Autodesk Fusion 360 part; units mm, degrees
note: some values were not read from the file. Chosen so that the rebuilt part matches the saved one: which pieces of a blend or face edit are solid. Set by a fixed rule: which sketch regions a step uses.
(part 3 of 3)
  dimension "d82" = 12
  dimension "d85" = 54
  dimension "d86" = 46.76
  dimension "d87" = 12
  dimension "d88" = 27
  dimension "d89" = 3
  dimension "d90" = -3
  dimension "d104" = 118
  dimension "d105" = 0
  dimension "d108" = 96
  dimension "d109" = 0
  dimension "d110" = 198
  dimension "d111" = 146
  constraint horizontal L0
  constraint vertical L1
  constraint horizontal L2
  constraint vertical L3
  constraint coincident L0.start L3.end
  constraint coincident L2.end L3.start
  constraint coincident L1.end L2.start
  constraint coincident L0.end L1.start
  constraint coincident L0 P0
  constraint midpoint L3 P6
  constraint midpoint L1 L4.end
  constraint coincident A0 L15.start
  constraint coincident A2 L16.end
  constraint parallel L2 L15
  constraint coincident A3 L17.start
  constraint coincident A1 L18.end
  constraint parallel L0 L17
  constraint concentric A4 A5
  constraint tangent A5 L15
  constraint coincident P6 P1
  constraint horizontal L6
  constraint horizontal L8
  constraint coincident L3 P8
  constraint coincident P8 P3
  constraint horizontal L10
  constraint perpendicular L14 L17
  constraint concentric A1 A6
  constraint concentric A0 A7
  constraint concentric A3 A8
  constraint concentric A2 A9
  constraint collinear L15 L16
  constraint collinear L17 L18
  constraint tangent L13 A10
  constraint tangent L20 A10
  constraint tangent L11 A11
  constraint tangent L19 A11
  constraint tangent L19 A12
  constraint tangent L14 A12
  constraint tangent L20 A13
  constraint tangent L12 A13
  constraint vertical L12
  constraint vertical L11
  constraint horizontal L19
  constraint horizontal L20
  constraint vertical L13
  constraint horizontal L33
  constraint horizontal L45
  constraint horizontal L36
  constraint horizontal L51
  constraint coincident L3 P10
  constraint horizontal L57
  constraint coincident A7 L58.start
  constraint coincident L2 L58.start
  constraint coincident A6 L58.end
  constraint coincident L0 L58.end
  constraint coincident A9 L59.start
  constraint coincident L2 L59.start
  constraint coincident A8 L59.end
  constraint coincident L0 L59.end
  constraint coincident L2 A4.centre
  constraint coincident A5 L15.end
  constraint coincident A5 L13.start
  constraint tangent A5 L13
  constraint coincident L12.start A18
  constraint coincident L18.start A18
  constraint tangent L18 A14
  constraint tangent L11 A16
  constraint coincident L11.start A16
  constraint coincident L14.end A27
  constraint tangent L14 A27
  constraint tangent L12 A18
  constraint perpendicular L1252 L1554
  measures "d1" distance of L0.start L0.end
  measures "d10" diameter of A0
  measures "d11" diameter of A1
  measures "d12" diameter of A2
  measures "d13" diameter of A3
  measures "d16" diameter of A4
  measures "d17" distance of L2 L15
  measures "d18" distance of L0 L17
  measures "d26" angle of L5 L6
  measures "d29" angle of L7 L8
  measures "d31" angle of L9 L10
  measures "d34" distance of P6 P8
  measures "d43" diameter of A6
  measures "d44" diameter of A7
  measures "d45" diameter of A8
  measures "d46" diameter of A9
  measures "d48" radius of A10
  measures "d49" radius of A11
  measures "d50" radius of A12
  measures "d51" radius of A13
  measures "d65" distance of L19 L20
  measures "d66" distance of L4 L19
  measures "d78" distance of L5 P8
  measures "d79" distance of P6 L33
  measures "d81" distance of P8 L45
  measures "d87" distance of P10 L57
  measures "d88" distance of P6 P10
  measures "d110" distance of A4.centre A24.centre
  measures "d111" distance of A4.centre L2.end
extrude "Extrude1" add sketch "Sketch1" along normal blind 14 contours A0 A7 L53 L54 L55 L257 L258 | A0 A1 A5 A14 A18 L21 A20 L22 A21 L23 L24 L25 L28 L29 L30 L33 L43 L44 L45 L46 L49 L50 L51 L52 L53 L57 L61 L70 L72 L73 L77 L78 L79 L81 L82 L90 L91 L92 L257 L260 L261 L263 L310 L312 L313 L314 L316 L317 L318 L319 L320 L321 L322 L323 L324 L330 L331 L332 L333 L334 L342 L346 L482 L483 L484 L492 L493 L494 L495 L496 L497 L501 L502 L503 L511 L512 L513 L514 L521 L522 L523 L525 L527 L528 L529 L530 L531 L532 L533 L540 L541 L542 L543 L544 L545 L549 L550 L551 L559 L560 L561 L562 L563 L564 L565 L568 L569 L570 L571 L733 L734 L781 L782 | A0 L257 L258 | A0 L53 L54 L61 | A0 L57 L58 L61 | A0 L54 L58 L61 | A0 L15 L24 L258 | L15 L24 L258 L260 | A0 A7 L54 L55 L58 | L30 L57 L58 L61 | L15 L24 L260 L484 | L30 L33 L58 L61 | L15 L24 L482 L484 | L24 L482 L483 L484 | L33 L45 L58 L61 | L15 L24 L482 L492 | A1 L45 L58 L61 | L15 L24 L492 L496 | A1 L42 L58 L61 | A1 L42 L43 L61 | L15 L24 L496 L497 | A1 A6 L41 L42 L58 | A1 A6 L41 L42 L43 L46 L47 | L15 L24 L497 L501 | L24 L497 L501 L503 | L15 L24 L501 L502 | A1 L18 L25 L47 | A1 L46 L47 | L15 L24 L502 L514 | L18 L25 L47 L49 | L15 L24 L514 L733 | L18 L25 L49 L77 | A5 L15 L24 L733 | A5 L24 L733 L734 | L18 L25 L73 L77 | A5 L734 L735 | L25 L72 L73 L77 | L18 L25 L73 L79 | A4 A5 L523 L524 L734 L735 L748 L749 | L18 L25 L79 L81 | A4 A5 L21 L523 L524 | L18 L25 L81 L90 | A5 L748 L749 | A5 L21 L524 | A5 L13 L21 L524 L525 | L18 L25 L90 L92 | A5 L13 L748 | A5 L13 L524 L748 | L13 A10 L21 A20 L525 L526 L529 L530 L535 L539 L540 | L25 L90 L91 L92 | L18 L25 L92 L316 | L21 A20 L529 L530 | L18 L25 L314 L316 | L13 L526 L535 | L18 L25 L314 L324 | L18 A14 L25 L324 | L20 A10 A20 L22 L539 L540 L544 | A14 L25 L323 L324 | L18 A14 L328 | A14 L25 L328 | A14 L25 L323 L328 | L18 A14 L25 L328 L329 | A14 L25 L328 | L20 L22 L544 L545 | A14 A15 L25 L320 L321 L323 L328 L329 L330 | L18 L25 L329 L333 | L20 L22 L545 L549 | A14 A15 L320 L321 | L18 L25 L333 L334 | A14 L329 L330 | L20 L22 L549 L550 | L18 L25 L334 L346 | L20 L22 L550 L562 | L18 L25 L346 L565 | L25 L334 L342 L346 | L20 L22 A21 L562 L781 | L18 A18 L25 L565 L567 | L18 A18 L567 L581 | L20 A13 A21 L781 L782 | L18 A18 L581 | A18 A19 L567 L568 L569 L575 L576 L581 | A18 L25 L567 | A18 L25 L567 L568 | L12 A13 A21 L23 L571 L782 | A18 L576 L581 | A18 A19 L569 L575 | L12 A18 L23 L571 picked at (-6.11229, 80.063542) picked at (175.409304, 31.163565) picked at (9.778758, 79.397633) picked at (7.933632, 74.992287) picked at (4, 58.820203) picked at (5, 75.333333) picked at (10.599079, 82.625193) picked at (19.628119, 82.333333) picked at (-5.975861, 75.691901) picked at (5, 53) picked at (36.26968, 83.166667) picked at (5, 35) picked at (49.167417, 83.166667) picked at (44.450599, 81.330232) picked at (4, 26) picked at (55.618076, 82.333333) picked at (4, 19.179797) picked at (66.3917, 82.333333) picked at (5, 2.666667) picked at (7.933632, 3.007713) picked at (84.667296, 82.333333) picked at (-5.975861, 2.308099) picked at (-6.11229, -2.063542) picked at (91.117955, 83.166667) picked at (91.215971, 81.330232) picked at (104.019273, 83.166667) picked at (10.599079, -4.625193) picked at (9.779197, -1.402707) picked at (113.157072, 82.333333) picked at (19.629909, -4.333333) picked at (131.429086, 82.333333) picked at (36.276842, -5.166667) picked at (135.442209, 82.541972) picked at (135.774404, 81.215707) picked at (49.170998, -5.166667) picked at (146.135399, 82.977036) picked at (44.455971, -3.333333) picked at (55.618076, -4.333333) picked at (149.896231, 77.792737) picked at (66.395281, -4.333333) picked at (148.132043, 74.135815) picked at (84.678039, -4.333333) picked at (150.909828, 80.139556) picked at (149.702921, 73.587232) picked at (150.333333, 64.44664) picked at (91.125117, -5.166667) picked at (151.864694, 76.222378) picked at (151.66289, 73.358797) picked at (151.166667, 58.828347) picked at (95.840145, -3.333333) picked at (102.381657, -4.333333) picked at (153.210199, 38.425578) picked at (113.157072, -4.333333) picked at (151.272341, 52.490696) picked at (131.443411, -4.333333) picked at (135.452953, -4.541972) picked at (168.596866, 34.833333) picked at (135.784085, -3.225963) picked at (148.44301, -5.712236) picked at (147.961885, -4.878902) picked at (145.285286, -3.334884) picked at (150.408509, -5.531332) picked at (148.457669, -4.647389) picked at (172.809437, 35.666667) picked at (149.900039, 0.194164) picked at (167.429787, -4.333333) picked at (183.397773, 35.666667) picked at (148.759831, 3.822414) picked at (178.208783, -4.333333) picked at (150.910613, -2.147933) picked at (201.302794, 35.666667) picked at (189.463532, -5.166667) picked at (212.938862, 34.833333) picked at (195.907029, -4.333333) picked at (189.368202, -3.334884) picked at (219.573018, 35.666667) picked at (206.011142, -4.333333) picked at (222.378448, -5.338127) picked at (222.749908, 35.617912) picked at (225.276189, -5.974051) picked at (224.39213, -3.81012) picked at (222.490943, -4.235424) picked at (222.706004, -2.592618) picked at (230.333333, 25.663565) picked at (227.183872, -4.892286) picked at (228.47065, 4.015156) picked at (230.333333, 17.618263) makes body 1
extrude "Extrude2" add sketch "Sketch1" along normal blind 14 separate body contours L19 A11 A22 L63 L780 L784 | A11 A22 L770 L780 | L11 A11 L62 A22 L769 L770 | A16 L26 L27 L60 L62 A22 L63 A23 L64 A25 A27 L769 L770 L774 L775 L776 L777 L778 L779 L780 L784 L785 L786 L787 L788 L789 L790 L798 L802 L814 L822 L824 L825 L826 L827 L832 L833 L834 L835 L836 L837 L838 L846 L850 L986 L987 L996 L997 L998 L999 L1000 L1001 L1005 L1006 L1007 L1015 L1016 L1017 L1018 L1019 L1020 L1021 L1023 L1024 L1032 L1033 L1034 L1035 L1036 L1037 L1067 L1068 L1069 L1071 L1072 L1078 L1080 L1081 L1085 L1086 L1087 L1089 L1090 L1098 L1099 L1100 L1237 L1238 L1239 L1249 L1250 L1251 L1252 L1253 L1255 L1256 L1257 L1265 L1266 L1268 L1269 L1271 L1313 L1314 L1324 L1325 L1490 L1491 L1492 L1500 L1501 L1502 L1503 L1504 L1505 L1509 L1510 L1511 L1519 L1524 L1525 | L19 L63 L784 L785 | L11 L62 L769 L775 | L19 L63 L785 L789 | L11 L62 L766 L775 | L19 L63 L789 L790 | L11 A16 L62 L765 L766 | L19 L63 L790 L802 | L11 A16 L765 | A16 L62 L766 | L19 L63 L802 L1021 | A16 L764 L765 | A16 L62 L765 | A16 A17 L62 L764 L765 L766 L774 L987 L988 | A16 A17 L766 L774 | L19 A12 L63 A23 L1021 L1022 L1023 | A16 L27 L988 | L14 A12 A23 L64 L812 L813 L814 L1022 L1023 L1036 L1037 | L16 A16 L27 L986 | A16 L27 L987 L988 | A16 L27 L986 L987 | L16 L27 L986 L996 | L14 L812 L813 | A23 L64 L1036 L1037 | L16 L27 L996 L1000 | L16 L27 L1000 L1001 | L14 L64 A27 L814 L823 | L16 L27 L1001 L1005 | L14 A27 L817 L823 | L16 L27 L1005 L1006 | L27 L1001 L1005 L1007 | L14 A27 L817 | A26 A27 L817 L818 L823 L824 L827 L828 | L64 A27 L823 | L64 A26 A27 L823 L824 | L16 L27 L1006 L1018 | A27 L817 L818 | L16 L27 L1018 L1237 | L16 L27 L1237 L1239 | A27 L827 L828 | L26 A27 L827 L832 | L16 L27 L1239 L1253 | L27 L1237 L1238 L1239 | L17 L26 A27 L832 | L16 L27 A25 L1253 | L17 L26 L832 L833 | L16 L27 A25 L1249 | L27 A25 | L27 A25 L1252 L1253 | L17 L26 L833 L837 | L16 L27 L1249 L1255 | L27 A25 L1252 | L27 A25 L1553 | L17 L26 L837 L838 | L16 L27 L1255 L1257 | A25 L1252 | L17 L26 L838 L850 | L26 L838 L846 L850 | L16 L27 L1257 L1266 | L27 L1255 L1256 L1257 | A25 L1252 L1554 | L17 L26 L850 L1069 | L16 L27 L1266 L1268 | L17 L26 L1069 L1071 | L16 L27 L1268 L1492 | L17 L26 L1071 L1085 | L16 L27 L1490 L1492 | L17 L26 L1081 L1085 | L26 L1080 L1081 L1085 | L16 L27 L1490 L1500 | L27 L1490 L1491 L1492 | L17 L26 L1081 L1087 | L16 L27 L1500 L1504 | L17 L26 L1087 L1089 | L16 L27 L1504 L1505 | L17 L26 L1089 L1098 | L16 L27 L1505 L1509 | L17 L26 L1098 L1100 | L26 L1098 L1099 L1100 | L16 L27 L1509 L1510 | L27 L1505 L1509 L1511 | L17 L26 L1100 L1324 | A2 L16 L27 L1510 | A3 L17 L26 L1324 | A3 L26 L60 L1324 L1325 | A2 | A2 L27 L60 L1510 L1519 | A3 | A3 L59 L60 L1320 L1325 | L59 L60 L1313 L1319 L1320 L1325 | A2 L59 L60 L1519 L1520 | L59 L60 L1519 L1520 L1523 L1524 | L59 L60 L1313 L1314 L1315 L1319 | L59 L60 L1523 L1524 L1525 L1526 | L59 L60 L1314 L1315 L1525 L1526 picked at (240.334724, 42.333333) picked at (223.22752, 45.338574) picked at (220.833333, 55.670564) picked at (223.963533, 57.05587) picked at (248.05205, 42.333333) picked at (221.666667, 59.034158) picked at (254.69695, 43.166667) picked at (221.666667, 66.007755) picked at (267.98675, 43.166667) picked at (220.833333, 69.494553) picked at (276.930307, 42.333333) picked at (220.708473, 73.75994) picked at (223.160749, 71.830131) picked at (293.179806, 43.166667) picked at (222.281583, 78.219094) picked at (221.815094, 74.842155) picked at (223.258231, 75.236965) picked at (225.158818, 73.36066) picked at (299.150792, 43.166667) picked at (227.001287, 83.075443) picked at (316.833333, 19.771431) picked at (238.134749, 82.333333) picked at (228.116601, 81.327131) picked at (237.629901, 81.213143) picked at (244.315389, 83.166667) picked at (316.607755, 25.486044) picked at (314.540637, 39.702424) picked at (253.449606, 82.333333) picked at (270.082214, 83.166667) picked at (317.666667, 13.953212) picked at (282.990695, 83.166667) picked at (316.267565, 4.095355) picked at (291.080761, 83.166667) picked at (282.890888, 81.327131) picked at (316.076333, 1.310426) picked at (317.937429, 0.003905) picked at (318.158468, 4.077407) picked at (319.583407, 3.526062) picked at (300.214978, 82.333333) picked at (316.850928, -1.850259) picked at (316.845795, 83.166667) picked at (329.754276, 83.166667) picked at (319.78146, -4.62039) picked at (331.974842, -3.231092) picked at (336.210307, 82.333333) picked at (329.653574, 81.32558) picked at (332.305449, -4.541972) picked at (339.054767, 82.541972) picked at (336.194191, -4.333333) picked at (358.319413, 82.333333) picked at (345.253104, 81.892093) picked at (337.750223, 80.324153) picked at (354.487693, -4.333333) picked at (363.607586, 83.166667) picked at (340.208322, 75.873434) picked at (349.228141, 81.318612) picked at (363.634445, -5.166667) picked at (376.519648, 83.166667) picked at (339.00265, 75.450039) picked at (376.517857, -5.166667) picked at (371.805516, -3.337985) picked at (382.975679, 82.333333) picked at (376.418946, 81.32558) picked at (341.27419, 72.479258) picked at (382.957773, -4.333333) picked at (393.743931, 82.333333) picked at (401.251275, -4.333333) picked at (410.371167, 83.166667) picked at (410.399816, -5.166667) picked at (423.283229, 83.166667) picked at (423.279648, -5.166667) picked at (423.187004, -3.339536) picked at (429.74105, 82.333333) picked at (423.181632, 81.324029) picked at (429.719563, -4.333333) picked at (440.507512, 82.333333) picked at (440.503931, -4.333333) picked at (457.132957, 83.166667) picked at (457.165188, -5.166667) picked at (470.048601, 83.166667) picked at (470.045019, -5.166667) picked at (469.952376, -3.339536) picked at (476.506422, 82.333333) picked at (469.947004, 81.324029) picked at (476.483144, -4.333333) picked at (479.581758, 82.333333) picked at (479.563852, -4.333333) picked at (478.568078, -2.384954) picked at (484.255191, 83.049067) picked at (478.576136, 80.367896) picked at (484.255191, -5.049067) picked at (485.67961, 10.031337) picked at (486.03159, 11.476739) picked at (485.678714, 67.934547) picked at (486.030695, 65.472087) picked at (486, 21.531456) picked at (486, 48.525253) picked at (485.062286, 39.473638) makes body 2
sketch "Sketch2" plane through (0, -6, 0) normal (0, -1, 0) x (1, 0, 0)
  line L0 (8, 0) -> (226, 0)
  line L1 (226, 0) -> (226, 14)
  line L2 (226, 14) -> (8, 14)
  line L3 (8, 14) -> (8, 0)
  circle A0 centre (328.140012, 4.999995) radius 2.175
  line L4 (324.965012, 4.999995) -> (324.965012, 0)
  circle A1 centre (220.334997, 4.999999) radius 2.175
  line L5 (217.159997, 0) -> (223.509997, 0)
  circle A2 centre (220.334997, 4.999999) radius 1.699995 construction
  line L6 (223.509997, 4.999999) -> (223.509997, 0)
  circle A3 centre (220.334997, 4.999999) radius 3.175
  line L7 (217.159997, 0) -> (217.159997, 4.999999)
  circle A4 centre (328.140012, 4.999995) radius 3.175
  line L8 (331.315012, 4.999995) -> (331.315012, 0)
  circle A5 centre (328.140012, 4.999995) radius 1.700004 construction
  line L9 (324.965012, 0) -> (331.315012, 0)
  point P0 (327.341034, 3.499446)
  point P1 (219.536049, 6.500554)
  point P2 (327.051003, 6.305397)
  point P3 (221.999046, 5.347739)
  point P4 (219.694569, 3.425249)
  point P5 (329.80407, 5.347739)
  dimension "d117" = 1
  dimension "d118" = 1
  dimension "d119" = 4.35
  dimension "d120" = 4.35
  dimension "d121" = 107.805015
  dimension "d122" = 5
  dimension "d123" = 5
  constraint concentric A1 A2
  constraint concentric A0 A5
  constraint tangent A3 L7
  constraint tangent L6 A3
  constraint tangent L4 A4
  constraint tangent A4 L8
  measures "d119" diameter of A1
  measures "d120" diameter of A0
extrude "Extrude3" add sketch "Sketch2" against normal blind 15 contours L0 L5 L6 A3 L7 | A3 | A0 | L4 A4 L8 L9 | A4 | A1 picked at (220.414086, 0.611292) picked at (223.156745, 4.734207) picked at (328.856914, 4.89194) picked at (328.219101, 0.611291) picked at (328.194191, 2.166275) picked at (220.988199, 4.685433) bodies 1 2
extrude "Extrude4" cut sketch "Sketch2" against normal blind 5 contours A0 | A1 picked at (328.856914, 4.89194) picked at (220.988199, 4.685433) bodies 1 2
chamfer "Chamfer2" distance 0.4 angle 45 4 faces at (219.781275, 2.081298, 0) (138.5348, 81.163565, 14) (481.096059, 73.598708, 0) (481.096059, 73.598708, 14) on bodies 1 2
chamfer "Chamfer2" distance 0.4 angle 45 2 edges at (218.307185, -6, 5.786512) (326.1122, -6, 5.786509) on bodies 1 2
equation "d18 = d17"
equation "d26 = ( ( 360 / 6 ) / 2 ) * 1 deg"
equation "d28 = ( 12 * 2 ) * 1 mm + 3 mm"
equation "d29 = 180 deg - d26"
equation "d31 = d26"
equation "d32 = d28"
equation "d66 = d65 / 2"
equation "d85 = ( 12 * 4 ) * 1 mm + ( 3 * 2 ) * 1 mm"
equation "d86 = ( 23.38 * 2 ) * 1 mm"
equation "d88 = d34"
equation "d111 = d1 / 2 - ( d110 / 2 )"
equation "d123 = d122"
